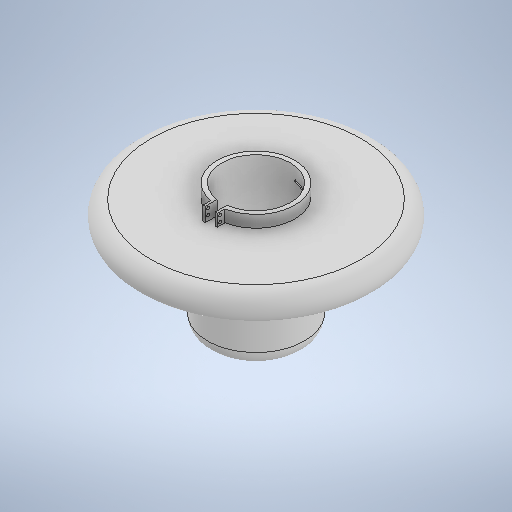
# Autodesk Inventor part: Water Sensor Bouy 3
Saved by Autodesk Inventor 2025 (Build 290162000, 162)
## iProperties
Created: 2024-06-24
Part Number: Water Sensor Bouy 3
Material: Generic
Document SubType Name: Modeling
Designer: track
Density: 1 g/cm^3
Appearance: Default
Mass: 228.42 g
Surface Area: 2248.19 cm^2
Volume: 228.42 cm^3
Author: track
## iProperties of the stored document Water Sensor Bouy 3_3DPrint.ipt
Created: 2024-06-24
Part Number: Water Sensor Bouy 3_3DPrint
Material: Generic
Document SubType Name: Modeling
Designer: track
Density: 1 g/cm^3
Appearance: Default
Author: track
Autodesk Inventor part; units mm, degrees
ref_plane "YZ Plane" through (0, 0, 0) normal (1, 0, 0) x (0, 1, 0)
sketch "Sketch2" plane through (0, 0, 0) normal (0, 0, 1) x (1, 0, 0)
  line L0 (0, 0) -> (0, 152.4)
  line L1 (30.98, 0) -> (30.98, 101.6)
  line L2 (30.98, 0) -> (30.98, 0)
  line L3 (43.68, 12.7) -> (43.68, 50.8)
  line L4 (69.08, 76.2) -> (94.48, 76.2)
  line L5 (107.18, 88.9) -> (107.18, 88.9)
  line L6 (94.48, 101.6) -> (30.98, 101.6)
  arc A0 (107.18, 88.9) -> (94.48, 101.6) centre (94.48, 88.9) ccw
  arc A1 (94.48, 76.2) -> (107.18, 88.9) centre (94.48, 88.9) ccw
  arc A2 (30.98, 0) -> (43.68, 12.7) centre (30.98, 12.7) ccw
  arc A3 (69.08, 76.2) -> (43.68, 50.8) centre (69.08, 50.8) ccw
  line L7 (41.68, 50.8) -> (41.68, 12.7)
  arc A4 (32.98, 2.1886) -> (41.68, 12.7) centre (30.98, 12.7) ccw
  line L8 (32.98, 2.1886) -> (32.98, 99.6)
  line L9 (32.98, 99.6) -> (94.48, 99.6)
  arc A5 (105.18, 88.9) -> (94.48, 99.6) centre (94.48, 88.9) ccw
  line L10 (105.18, 88.9) -> (105.18, 88.9)
  arc A6 (94.48, 78.2) -> (105.18, 88.9) centre (94.48, 88.9) ccw
  line L11 (94.48, 78.2) -> (69.08, 78.2)
  arc A7 (69.08, 78.2) -> (41.68, 50.8) centre (69.08, 50.8) ccw
  point P0 (43.68, 0)
  point P1 (43.68, 76.2)
  point P2 (107.18, 76.2)
  point P3 (107.18, 101.6)
  point P4 (89.9, 76.2)
  point P5 (105.18, 88.9)
  dimension "d0" = 30.98
  dimension "d1" = 101.6
  dimension "d2" = 152.4
  dimension "d3" = 76.2
  dimension "d4" = 12.7
  dimension "d5" = 25.4
  dimension "d7" = 76.2
  dimension "d9" = 90
  dimension "d10" = 0
  dimension "d11" = 12.7
  dimension "d12" = 25.4
  dimension "d48" = 2
  dimension "d49" = 2
  dimension "d50" = 2
  constraints: 24 end point, 16 point on circle, 8 centre point, 8 point on line, 8 tangent, 7 perpendicular, 2 equal radius, 2 vertical, 1 horizontal, 5 other
  measures "d0" distance between parallel lines of L0 L1
  measures "d1" distance of L1.start L1.end
  measures "d2" distance of L0.start L0.end
  measures "d3" distance of point (107.18, 101.6) L1.end
  measures "d4" distance between parallel lines of L1 L3
  measures "d5" distance of point (107.18, 76.2) point (107.18, 101.6)
  measures "d7" distance of point (43.68, 0) point (43.68, 76.2)
  measures "d9" angle of L1 L6
  measures "d10" distance from line of L0.start L2
  measures "d11" radius of A0
  measures "d12" radius of A3
  measures "d48" distance between parallel lines of L1 L8
  measures "d49" radial gap between concentric circles of A2 A4
  measures "d50" distance between parallel lines of L4 L11
revolve "Revolution1" add sketch "Sketch2" angle 360 about axis through (0, 0, 0) along (0, 1, 0)
ref_plane "Work Plane1" through (0, 38.1, 0) normal (0, -1, 0) x (1, 0, 0)
sketch "Sketch4" plane through (0, 38.1, 0) normal (0, -1, 0) x (1, 0, 0)
  circle A0 centre (0, 69.85) radius 3
  circle A1 centre (0, 0) radius 30.98 projected
  line L0 (0, 30.98) -> (0, 107.18)
  circle A2 centre (0, 0) radius 107.18 projected
  dimension "d18" = 76.2
  dimension "d19" = 6
  dimension "d20" = 69.85
  constraints: 2 end point, 2 vertical alignment, 1 centre point, 1 point on line, 1 vertical, 2 other
  measures "d18" distance of L0.start L0.end
  measures "d19" diameter of A0
  measures "d20" distance of point (0, 0) A0.centre
extrude "Extrusion1" cut sketch "Sketch4" against normal blind 50.8 contours A0 L0 | L0 A0
pattern_circular "Circular Pattern1" count 3 over 360 about axis through (0, 50.8, 0) along (0, 1, 0) of "Extrusion1"
sketch "Sketch5" plane through (0, 101.6, 0) normal (0, 1, 0) x (1, 0, 0)
  circle A0 centre (0, 0) radius 30.98
  circle A1 centre (0, 0) radius 34.98
  circle A2 centre (0, 0) radius 30.98 projected
  dimension "d26" = 4
  constraints: 2 centre point, 2 coincident, 1 concentric
  measures "d26" radial gap between concentric circles of A0 A1
extrude "Extrusion2" add sketch "Sketch5" along normal blind 12.7
ref_plane "Work Plane2" through (0, 101.6, 34.98) normal (0, 0, 1) x (1, 0, 0)
sketch "Sketch6" plane through (0, 101.6, 34.98) normal (0, 0, 1) x (1, 0, 0)
  line L0 (94.48, 0) -> (-94.48, 0) projected
  line L1 (-30.98, 12.7) -> (30.98, 12.7) projected
  line L2 (-4.445, 0) -> (-6.445, 0)
  line L3 (-6.445, 0) -> (-6.445, 12.7)
  line L4 (-6.445, 12.7) -> (-4.445, 12.7)
  line L5 (-4.445, 12.7) -> (-4.445, 0)
  line L6 (4.445, 0) -> (6.445, 0)
  line L7 (6.445, 0) -> (6.445, 12.7)
  line L8 (6.445, 12.7) -> (4.445, 12.7)
  line L9 (4.445, 12.7) -> (4.445, 0)
  line L10 (0, 12.7) -> (0, 0)
  point P0 (0, -101.6)
  point P1 (-6.445, 0)
  point P2 (4.445, 12.7)
  point P3 (4.445, 0)
  point P4 (6.445, 0)
  point P5 (6.445, 12.7)
  dimension "d30" = 2
  dimension "d31" = 8.89
  constraints: 18 end point, 4 parallel, 4 point on line, 2 horizontal, 2 midpoint, 2 perpendicular, 2 other
  measures "d30" distance between parallel lines of L9 L7
  measures "d31" distance between parallel lines of L5 L9
extrude "Extrusion3" add sketch "Sketch6" along normal blind 6.35 and the other way blind 1.27 contours L0 L9 L1 L7 | L0 L3 L1 L5
sketch "Sketch7" plane through (0, 101.6, 34.98) normal (0, 0, 1) x (1, 0, 0)
  line L0 (-4.445, 0) -> (4.445, 0) projected
  line L1 (4.445, 12.7) -> (-4.445, 12.7) projected
  line L2 (-4.445, 0) -> (4.445, 0)
  line L3 (4.445, 0) -> (4.445, 12.7)
  line L4 (4.445, 12.7) -> (-4.445, 12.7)
  line L5 (-4.445, 12.7) -> (-4.445, 0)
  point P0 (0, -101.6)
  constraints: 8 end point, 2 parallel, 1 horizontal, 1 perpendicular
extrude "Extrusion4" cut sketch "Sketch7" against normal up to surface round surface about axis through (0, 50.8, 0) along (0, 1, 0) radius 30.98 far side no
sketch "Sketch8" plane through (0, 101.6, 41.33) normal (0, 0, 1) x (1, 0, 0)
  line L0 (4.445, 0) -> (-4.445, 0) projected
  line L1 (34.98, 0) -> (34.98, 12.7) projected
  line L2 (4.445, 0) -> (34.98, 0)
  line L3 (34.98, 0) -> (34.98, 1.905)
  line L4 (34.98, 1.905) -> (4.445, 1.905)
  line L5 (4.445, 1.905) -> (4.445, 0)
  point P0 (0, -101.6)
  dimension "d38" = 1.905
  constraints: 8 end point, 2 parallel, 1 horizontal, 1 perpendicular, 1 point on line
  measures "d38" distance between parallel lines of L2 L4
extrude "Extrusion5" cut sketch "Sketch8" against normal blind 101.6
sketch "Sketch9" plane through (6.445, 114.3, 41.33) normal (1, 0, 0) x (0, 0, -1)
  line L0 (10.6705, 0) -> (0, 0) projected
  line L1 (2.54, 0) -> (2.54, -10.795)
  line L2 (0, -10.795) -> (6.9489, -10.795) projected
  line L3 (0, -10.795) -> (0, 0) projected
  circle A0 centre (2.54, -2.667) radius 1.3335
  circle A1 centre (2.54, -8.128) radius 1.3335
  point P0 (41.33, -114.3)
  dimension "d41" = 2.54
  dimension "d42" = 2.667
  dimension "d43" = 2.667
  dimension "d44" = 2.667
  dimension "d45" = 2.667
  constraints: 4 point on line, 2 centre point, 2 end point, 1 vertical
  measures "d41" distance between parallel lines of L3 L1
  measures "d42" diameter of A0
  measures "d43" diameter of A1
  measures "d44" distance from line of L2 A1.centre
  measures "d45" distance from line of L0 A0.centre
extrude "Extrusion6" cut sketch "Sketch9" against normal up to surface (12.89 mm away) contours A0 L1 | L1 A0 | A1 L1 | L1 A1
body "Solid1"
